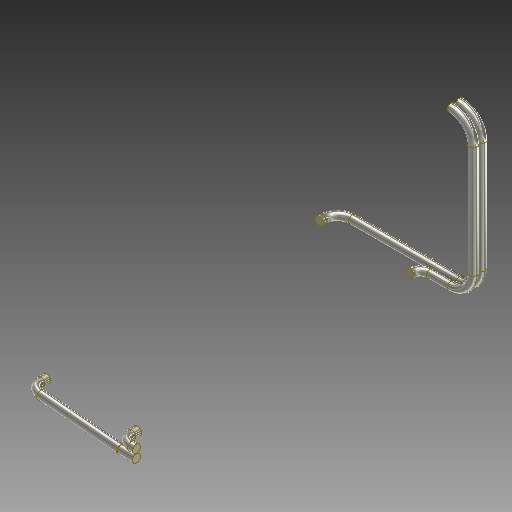
# Autodesk Inventor part: HVU_wires_resistor_WHS7
Saved by Autodesk Inventor 2017 (Build 210142000, 142)
## iProperties
Part Number: HVU_wires_resistor_WHS7
Material: Silber
Document SubType Name: Modeling
Designer: David
Density: 10.49 g/cm^3
Appearance: Silber
Author: David
Autodesk Inventor part; units mm, degrees
sketch "Skizze1" plane through (0, 0, 0) normal (0, 0, 1) x (1, 0, 0)
  line L0 (83.5734, 13.4619) -> (82.7634, 13.4619) projected
  line L1 (92.5734, 13.4619) -> (91.7634, 13.4619) construction
  line L2 (92.1684, 13.4619) -> (92.1684, 13.4619)
  line L3 (93.1684, 14.4619) -> (95.2684, 14.4619)
  arc A0 (93.1684, 14.4619) -> (92.1684, 13.4619) centre (93.1684, 13.4619) ccw
  line L4 (97.0184, -63.0081) -> (97.0184, 45.2749) construction
  point P0 (0, 0)
  dimension "d0" = 1
  dimension "d1" = 1.75
  dimension "d2" = 1
  constraints: 6 end point, 2 perpendicular, 2 point on circle, 2 tangent, 1 centre point, 1 midpoint, 1 vertical, 2 other
  measures "d0" radius of A0
  measures "d1" distance from line of L3.end L4
  measures "d2" distance between parallel lines of L3 L1
ref_plane "Arbeitsebene1" through (92.1684, 13.4619, 0) normal (0, 1, 0) x (-1, 0, 0)
sketch "Skizze2" plane through (92.1684, 13.4619, 0) normal (0, 1, 0) x (-1, 0, 0)
  circle A0 centre (0, 0) radius 0.405 projected
  point P0 (92.1684, 0)
sweep "Sweeping1" add profiles "Skizze2" path "Skizze1" path curves L2 A0 L3
ref_plane "Arbeitsebene3" through (95.2684, 14.4619, 0) normal (0, 1, 0) x (-1, 0, 0)
ref_plane "Arbeitsebene2" through (92.1684, 12.4619, 0) normal (0, 1, 0) x (-1, 0, 0)
sketch "Skizze3" plane through (95.2684, 14.4619, 0) normal (0, 1, 0) x (-1, 0, 0)
  line L0 (0, 0.405) -> (0, -0.405) construction
  line L1 (0, 0) -> (0, 0) construction
  line L2 (-2.1442, 2.1442) -> (-2.1442, 13.1493)
  line L3 (0, 13.1493) -> (-1.7392, 13.1493) construction
  arc A0 (0, 15.2936) -> (-2.1442, 13.1493) centre (0, 13.1493) ccw
  arc A1 (-2.1442, 2.1442) -> (0, 0) centre (0, 2.1442) ccw
  circle A2 centre (0, 12.9556) radius 1.75 projected
  point P0 (95.2684, 0)
  dimension "d5" = 0.81
  dimension "d6" = 0.405
  constraints: 6 end point, 5 point on circle, 2 centre point, 2 horizontal, 2 tangent, 1 coincident, 1 equal radius, 1 midpoint, 1 point on line, 1 other
  measures "d5" distance of L0.start L0.end
  measures "d6" distance from line of L2 L3.end
sketch "Skizze4" plane through (95.2684, 14.4619, 0) normal (1, 0, 0) x (0, 0, -1)
  circle A0 centre (0, 0) radius 0.405 projected
  point P0 (0, -14.4619)
sweep "Sweeping2" add profiles "Skizze4" path "Skizze3" path curves A1 L2 A0
pattern_linear "Rechteckige Anordnung1" count 2 spacing 0.81 along (0, 1, 0) of "Sweeping2"
sketch "Skizze5" plane through (0, 0, 0) normal (0, 0, 1) x (1, 0, 0)
  line L0 (83.5734, 13.4619) -> (82.7634, 13.4619) construction
  line L1 (95.2684, 15.6769) -> (95.2684, 14.8669) construction
  line L2 (95.2684, 15.2719) -> (84.6684, 15.2719)
  line L3 (83.1684, 13.7719) -> (83.1684, 13.4619)
  arc A0 (84.6684, 15.2719) -> (83.1684, 13.7719) centre (84.6684, 13.7719) ccw
  point P0 (0, 0)
  dimension "d13" = 1.5
  constraints: 4 end point, 2 midpoint, 2 perpendicular, 2 point on circle, 2 tangent, 1 centre point
  measures "d13" radius of A0
sketch "Skizze6" plane through (92.1684, 13.4619, 0) normal (0, 1, 0) x (-1, 0, 0)
  circle A0 centre (9, 0) radius 0.405 projected
  point P0 (92.1684, 0)
sweep "Sweeping3" add profiles "Skizze6" path "Skizze5"
sketch "Skizze7" plane through (0, 0, 0) normal (0, 0, 1) x (1, 0, 0)
  line L0 (92.5734, -13.5381) -> (91.7634, -13.5381) construction
  line L1 (83.8684, -15.5381) -> (94.1684, -15.5381) construction
  line L2 (92.1684, -13.5381) -> (92.1684, -14.1331)
  line L3 (93.1684, -15.1331) -> (93.6684, -15.1331)
  arc A0 (92.1684, -14.1331) -> (93.1684, -15.1331) centre (93.1684, -14.1331) ccw
  line L4 (94.1684, -15.5381) -> (94.1684, -19.9981) construction
  point P0 (0, 0)
  dimension "d16" = 0.81
  dimension "d17" = 0.405
  dimension "d18" = 1
  dimension "d19" = 0.5
  constraints: 4 end point, 2 point on circle, 2 tangent, 1 centre point, 1 midpoint, 1 perpendicular, 1 vertical
  measures "d16" distance of L0.start L0.end
  measures "d17" distance from line of L1.end L3
  measures "d18" radius of A0
  measures "d19" distance from line of L3.end L4
ref_plane "Arbeitsebene4" through (92.1684, -13.5381, 0) normal (0, -1, 0) x (1, 0, 0)
sketch "Skizze8" plane through (92.1684, -13.5381, 0) normal (0, -1, 0) x (1, 0, 0)
  circle A0 centre (0, 0) radius 0.405 projected
  point P0 (-92.1684, 0)
sweep "Sweeping4" add profiles "Skizze8" path "Skizze7"
sketch "Skizze9" plane through (92.1684, -13.5381, 0) normal (0, -1, 0) x (1, 0, 0)
  circle A0 centre (-9, 0) radius 0.405 construction
  circle A1 centre (0, 0) radius 0.405 construction
  line L0 (-10.153, 0.5108) -> (1.4679, -0.5393) construction
  line L1 (0.0022, -0.0035) -> (-0.0364, -0.4034) construction
  line L2 (-9, 0) -> (-8.9635, 0.4034) construction
  line L3 (-0.0364, -0.4034) -> (-0.0729, -0.8067) construction
  line L4 (-0.0729, -0.8067) -> (-9, 0) construction
  point P0 (-92.1684, 0)
  constraints: 10 end point, 2 point on line, 1 parallel, 1 perpendicular, 6 other
ref_plane "Arbeitsebene6" through (92.0955, -13.5381, -0.8067) normal (0.09, 0, 0.9959) x (-0.9959, 0, 0.09)
ref_plane "Arbeitsebene5" through (92.1684, -12.5381, 0) normal (0, -1, 0) x (1, 0, 0)
sketch "Skizze10" plane through (92.0955, -13.5381, -0.8067) normal (0.09, 0, 0.9959) x (-0.9959, 0, 0.09)
  line L0 (8.5585, 0) -> (9.3685, 0) construction
  line L1 (8.9635, 0) -> (8.9635, 0.595)
  arc A0 (8.9635, 0.595) -> (7.9635, 1.595) centre (7.9635, 0.595) ccw
  line L2 (7.9635, 0.595) -> (8.9635, 0.595) construction
  line L3 (7.9635, 1.595) -> (7.9635, 0.595) construction
  line L4 (-0.405, 0) -> (0.405, 0) construction
  line L5 (0.405, 0.595) -> (-0.405, 0.595) construction
  line L6 (-0.405, 0) -> (0.405, 0) construction
  line L7 (0, 0.595) -> (0, 1.595) construction
  ellipse E0 centre (-0.9959, 1.595) end of major axis (-0.9959, 2) minor radius 0.0365 construction
  line L8 (0, 1.595) -> (7.9635, 1.595)
  point P0 (91.7944, -13.5381)
  dimension "d23" = 1
  constraints: 10 end point, 4 perpendicular, 2 midpoint, 2 point on circle, 1 centre point, 1 point on line, 1 vertical, 1 other
  measures "d23" distance of L2.start L3.start
sketch "Skizze11" plane through (92.1684, -13.5381, 0) normal (0, -1, 0) x (1, 0, 0)
  circle A0 centre (-9, 0) radius 0.405 projected
  point P0 (-92.1684, 0)
sweep "Sweeping5" add profiles "Skizze11" path "Skizze10"
ref_plane "Arbeitsebene8" through (92.0955, -15.1331, -0.8067) normal (0, -1, 0) x (1, 0, 0)
ref_plane "Arbeitsebene7" through (92.1684, -12.5381, 0) normal (0, -1, 0) x (1, 0, 0)
sketch "Skizze12" plane through (92.0955, -15.1331, -0.8067) normal (0, -1, 0) x (1, 0, 0)
  line L0 (1.5729, 0.4017) -> (1.5729, 1.2117) construction
  line L1 (1.0729, 0.4017) -> (1.5729, 0.4017) construction
  circle A0 centre (0.0729, 0.8067) radius 0.405 construction
  circle A1 centre (0.0729, 0.8067) radius 0.405 construction
  arc A2 (0, 0) -> (0.0729, -0.0033) centre (0.0729, 0.8067) ccw
  line L2 (1.5729, 0.8067) -> (1.5729, -0.0033) construction
  line L3 (1.5729, -0.0033) -> (0.0729, -0.0033)
  point P0 (-92.0955, 0.8067)
  dimension "d26" = 0.81
  dimension "d27" = 0.81
  constraints: 4 end point, 2 coincident, 2 point on circle, 1 centre point, 1 collinear, 1 midpoint, 1 tangent
  measures "d26" distance of L0.start L0.end
  measures "d27" distance of L2.start L2.end
sketch "Skizze13" plane through (92.0955, -15.1331, -0.8067) normal (0.9959, 0, -0.09) x (-0.09, 0, -0.9959)
  circle A0 centre (0, 0) radius 0.405 projected
  point P0 (7.4852, 15.1331)
sweep "Sweeping6" add profiles "Skizze13" path "Skizze12"
equation "\"d6\" = 0.5 * d5"
equation "\"d17\" = 0.5 * d16"
equation "\"d27\" = d26"
